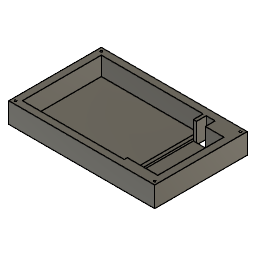
Case_bottom_source (Autodesk Fusion 360 design; units mm, degrees)
Autodesk Fusion 360 part; units mm, degrees
sketch "Sketch1" plane through (0, 0, 0) normal (0, 0, 1) x (1, 0, 0)
  line L0 (-50, 40) -> (143.2, 40)
  line L1 (143.2, 40) -> (143.2, -75.2)
  line L2 (143.2, -75.2) -> (-50, -75.2)
  line L3 (-50, -75.2) -> (-50, 40)
  line L4 (-60, 50) -> (153.2, 50)
  line L5 (153.2, 50) -> (153.2, -85.2)
  line L6 (153.2, -85.2) -> (-60, -85.2)
  line L7 (-60, -85.2) -> (-60, 50)
  circle A0 centre (-55, 45) radius 1.45
  circle A1 centre (148.2, 45) radius 1.45
  circle A2 centre (148.2, -80.2) radius 1.45
  circle A3 centre (-55, -80.2) radius 1.45
  line L8 (143.2, -75.2) -> (98.7, -75.2)
  line L9 (98.7, -75.2) -> (98.7, 21.3)
  line L10 (98.7, 21.3) -> (143.2, 21.3)
  line L11 (143.2, 21.3) -> (143.2, -75.2)
  line L12 (98.7, 21.3) -> (143.2, 21.3)
  line L13 (143.2, 21.3) -> (143.2, 40)
  line L14 (143.2, 40) -> (98.7, 40)
  line L15 (98.7, 40) -> (98.7, 21.3)
  line L16 (98.7, 40) -> (93.7, 40)
  line L17 (93.7, 40) -> (93.7, -75.2)
  line L18 (93.7, -75.2) -> (98.7, -75.2)
  line L19 (98.7, -75.2) -> (98.7, 40)
  dimension "d1" = 193.2
  dimension "d2" = 115.2
  dimension "d3" = 213.2
  dimension "d4" = 135.2
  dimension "d5" = 10
  dimension "d6" = 10
  dimension "d7" = 2.9
  dimension "d8" = 5
  dimension "d9" = 5
  dimension "d10" = 2.9
  dimension "d11" = 5
  dimension "d12" = 5
  dimension "d13" = 2.9
  dimension "d14" = 5
  dimension "d15" = 5
  dimension "d16" = 2.9
  dimension "d17" = 5
  dimension "d18" = 5
  dimension "d19" = 44.5
  dimension "d20" = 96.5
  dimension "d21" = 5
  constraint horizontal L0
  constraint vertical L1
  constraint horizontal L2
  constraint vertical L3
  constraint horizontal L4
  constraint vertical L5
  constraint horizontal L6
  constraint vertical L7
  constraint horizontal L8
  constraint vertical L9
  constraint horizontal L10
  constraint vertical L11
  constraint horizontal L12
  constraint vertical L13
  constraint horizontal L14
  constraint vertical L15
  constraint horizontal L16
  constraint vertical L17
  constraint horizontal L18
  constraint vertical L19
  measures "d1" distance of L0.start L0.end
  measures "d2" distance of L0.start L2.end
  measures "d3" distance of L4.start L4.end
  measures "d4" distance of L4.start L6.end
  measures "d5" distance of L3 L7
  measures "d6" distance of L0 L4
  measures "d7" diameter of A0
  measures "d8" distance of L4 A0.centre
  measures "d9" distance of L7 A0.centre
  measures "d10" diameter of A1
  measures "d11" distance of L4 A1.centre
  measures "d12" distance of L5 A1.centre
  measures "d13" diameter of A2
  measures "d14" distance of L6 A2.centre
  measures "d15" distance of L5 A2.centre
  measures "d16" diameter of A3
  measures "d17" distance of L6 A3.centre
  measures "d18" distance of L7 A3.centre
  measures "d19" distance of L1.end L8.end
  measures "d20" distance of L1.end L10.end
  measures "d21" distance of L14.end L16.end
extrude "Extrude1" add sketch "Sketch1" along normal blind 3 contours L0 L2 L3 L17 | L1 L2 L8 L9 L10 L11 L12 L19 makes body 1 at (113.5333, -43.0333, 0) makes body 2 at (-2.1, 1.6, 0)
extrude "Extrude2" add sketch "Sketch1" along normal blind 6 contours L0 L2 L9 L15 L16 L17 L18 L19 bodies 1 2
extrude "Extrude3" add sketch "Sketch1" along normal blind 3 separate body contours A0 | A1 | A2 | A3 makes body 3 at (149.5361, -79.6368, 2) makes body 4 at (-54.0406, -79.1128, 2) makes body 5 at (149.3558, 45.8755, 2) makes body 6 at (-56.4213, 45.2873, 2)
extrude "Extrude4" add sketch "Sketch1" along normal blind 30 contours L0 L1 L10 L12 L13 L14 L15 L19 | L4 L5 L6 L7 bodies 1 3 4 5 6
sketch "Sketch2" plane through (0, 21.3, 0) normal (0, -1, 0) x (1, 0, 0)
  line L0 (98.7, 3) -> (143.2, 3)
  line L1 (143.2, 3) -> (143.2, 30)
  line L2 (143.2, 30) -> (98.7, 30)
  line L3 (98.7, 30) -> (98.7, 6)
  line L4 (98.7, 6) -> (98.7, 3)
  line L5 (103.2, 30) -> (116.2, 30)
  line L6 (116.2, 30) -> (116.2, 3)
  line L7 (116.2, 3) -> (103.2, 3)
  line L8 (103.2, 3) -> (103.2, 30)
  dimension "d30" = 13
  dimension "d32" = 4.5
  constraint horizontal L5
  constraint vertical L6
  constraint horizontal L7
  constraint vertical L8
  constraint coincident L0 L6.end
  constraint coincident L2 L5.start
  measures "d30" distance of L5.start L5.end
  measures "d32" distance of L3 L8
extrude "Extrude5" cut sketch "Sketch2" against normal blind 18.7 contours L0 L2 L5 L6 L7 L8 bodies 1
sketch "Sketch3" plane through (0, 0, 3) normal (0, 0, 1) x (-1, 0, 0)
  line L0 (-98.7, 75.2) -> (-143.2, 75.2)
  line L1 (-143.2, 75.2) -> (-143.2, -21.3)
  line L2 (-143.2, -21.3) -> (-116.2, -21.3)
  line L3 (-116.2, -21.3) -> (-116.2, -40)
  line L4 (-116.2, -40) -> (-103.2, -40)
  line L5 (-103.2, -40) -> (-103.2, -21.3)
  line L6 (-103.2, -21.3) -> (-98.7, -21.3)
  line L7 (-98.7, -21.3) -> (-98.7, 75.2)
  line L8 (-103.2, -40) -> (-116.2, -40)
  line L9 (-116.2, -40) -> (-116.2, -21.3)
  line L10 (-116.2, -21.3) -> (-103.2, -21.3)
  line L11 (-103.2, -21.3) -> (-103.2, -40)
  constraint horizontal L8
  constraint vertical L9
  constraint horizontal L10
  constraint vertical L11
  constraint coincident L2.end L3.start
  constraint coincident L4.end L5.start
extrude "Extrude6" cut sketch "Sketch3" against normal blind 6 contours L3 L4 L5 L8 L9 L10 L11 bodies 1
sketch "Sketch4" plane through (0, -75.2, 0) normal (0, 1, 0) x (-1, 0, 0)
  line L0 (-143.2, 3) -> (-98.7, 3)
  line L1 (-98.7, 3) -> (-98.7, 6)
  line L2 (-98.7, 6) -> (-93.7, 6)
  line L3 (-93.7, 6) -> (-93.7, 3)
  line L4 (-93.7, 3) -> (50, 3)
  line L5 (50, 3) -> (50, 30)
  line L6 (50, 30) -> (-143.2, 30)
  line L7 (-143.2, 30) -> (-143.2, 3)
  line L8 (-98.7, 3) -> (-143.2, 3)
  line L9 (-143.2, 3) -> (-143.2, 30)
  line L10 (-143.2, 30) -> (-98.7, 30)
  line L11 (-98.7, 30) -> (-98.7, 3)
  constraint horizontal L8
  constraint vertical L9
  constraint horizontal L10
  constraint vertical L11
  constraint coincident L6.end L7.start
  constraint coincident L0.end L1.start
extrude "Extrude7" add sketch "Sketch4" along normal blind 4.5 contours L0 L1 L6 L7 L8 L9 L10 L11 bodies 1
extrude "Extrude8" cut 2 faces at (101.7, 21.3, 13) (125.2, 21.3, 12) along direction (0, 1, 0) blind 4.5 on bodies 1 bodies 1
extrude "Extrude9" add 1 faces at (111.8667, 21.3, 2) along direction (0, 1, 0) blind 4.5 on bodies 1 bodies 1
equation "d3 = 193.2 mm + 20 mm"
equation "d4 = 115.2 mm + 20 mm"
